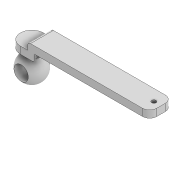
# Autodesk Inventor part: VentilNukleator2
Saved by Autodesk Inventor 2021 (Build 250183000, 183)
## iProperties
Created: 2022-03-14
Part Number: VentilNukleator2
Material: Generisch
Document SubType Name: Modeling
Designer: lukas
Density: 1 g/cm^3
Appearance: Vorgabe
Author: lukas
Autodesk Inventor part; units mm, degrees
ref_plane "YZ Plane" through (0, 0, 0) normal (1, 0, 0) x (0, 1, 0)
ref_plane "XY Plane" through (0, 0, 0) normal (0, 0, 1) x (1, 0, 0)
sketch "Skizze4" plane through (0, 0, 0) normal (0, 0, 1) x (1, 0, 0)
  line L0 (-12.6, 0) -> (12.6, 0) projected
  line L1 (0, -12.6) -> (0, 12.6) projected
  circle A0 centre (0, 0) radius 9
  point P0 (-9, 0)
  point P1 (9, 0)
  dimension "d8" = 18
  constraints: 1 centre point, 1 coincident
  measures "d8" diameter of A0
revolve "Umdrehung1" add sketch "Skizze4" angle 360 about axis through (-10, 0, 0) along (1, 0, 0) picked at (-5.0484, 3.1721) picked at (5.9248, 0.6676) contours A0 L1 L0 | L1 A0 L0
ref_plane "Arbeitsebene1" through (0, 9, 0) normal (0, 1, 0) x (-1, 0, 0)
sketch "Skizze5" plane through (0, 9, 0) normal (0, 1, 0) x (-1, 0, 0)
  circle A0 centre (0, 0) radius 2.5
  dimension "d11" = 5
  constraints: 1 centre point, 1 coincident
  measures "d11" diameter of A0
extrude "Extrusion3" add sketch "Skizze5" along normal mid plane 1
sketch "Skizze6" plane through (0, 9.5, 0) normal (0, 1, 0) x (1, 0, 0)
  circle A0 centre (0, 0) radius 2.5 projected
  circle A1 centre (0, 0) radius 2.5
  dimension "d14" = 5
  constraints: 1 centre point, 1 coincident
  measures "d14" diameter of A1
extrude "Extrusion4" add sketch "Skizze6" along normal blind 2
sketch "Skizze7" plane through (0, 0, 0) normal (0, 0, 1) x (1, 0, 0)
  circle A0 centre (0, 0) radius 5
  dimension "d17" = 10
  constraints: 1 centre point, 1 coincident
  measures "d17" diameter of A0
extrude "Extrusion5" cut sketch "Skizze7" along normal mid plane 20
sketch "Skizze8" plane through (0, 11.5, 0) normal (0, 1, 0) x (1, 0, 0)
  circle A0 centre (0, 0) radius 7.9569
  dimension "d20" = 15.9138
  constraints: 1 centre point, 1 coincident
  measures "d20" diameter of A0
extrude "Extrusion6" add sketch "Skizze8" along normal blind 5
sketch "Skizze9" plane through (0, 0, 0) normal (1, 0, 0) x (0, 1, 0)
  line L0 (16.5, -7.9569) -> (16.5, 7.9569) projected
  line L1 (11.5, -7.9569) -> (11.5, 7.9569) projected
  line L2 (16.5, 7.9569) -> (11.5, 7.9569)
  line L3 (11.5, 7.9569) -> (11.5, -7.9569)
  line L4 (11.5, -7.9569) -> (16.5, -7.9569)
  line L5 (16.5, -7.9569) -> (16.5, 7.9569)
  point P0 (0, 0)
  constraints: 8 end point, 2 parallel, 1 horizontal, 1 perpendicular
extrude "Extrusion7" add sketch "Skizze9" along normal blind 10
sketch "Skizze10" plane through (0, 16.5, 0) normal (0, 1, 0) x (1, 0, 0)
  line L0 (10, 7.9569) -> (10, -7.9569) projected
  line L1 (0, 7.9569) -> (10, 7.9569) projected
  line L2 (10, -7.9569) -> (5, -7.9569)
  line L3 (5, -7.9569) -> (5, 7.9569)
  line L4 (5, 7.9569) -> (10, 7.9569)
  line L5 (10, 7.9569) -> (10, -7.9569)
  point P0 (0, 0)
  dimension "d25" = 5
  constraints: 8 end point, 2 parallel, 1 horizontal, 1 midpoint, 1 perpendicular
  measures "d25" distance between parallel lines of L3 L0
extrude "Extrusion8" add sketch "Skizze10" along normal blind 5
sketch "Skizze11" plane through (10, 0, 0) normal (1, 0, 0) x (0, 0, -1)
  line L0 (7.9569, 11.5) -> (7.9569, 21.5) projected
  line L1 (-7.9569, 11.5) -> (-7.9569, 21.5) projected
  line L2 (7.9569, 21.5) -> (-7.9569, 21.5)
  line L3 (-7.9569, 21.5) -> (-7.9569, 16.5)
  line L4 (-7.9569, 16.5) -> (7.9569, 16.5)
  line L5 (7.9569, 16.5) -> (7.9569, 21.5)
  point P0 (0, 0)
  point P1 (7.9569, 16.5)
  dimension "d28" = 5
  constraints: 8 end point, 2 parallel, 1 horizontal, 1 midpoint, 1 perpendicular
  measures "d28" distance between parallel lines of L4 L2
extrude "Extrusion9" add sketch "Skizze11" along normal blind 80
fillet "Rundung2" radius 2 2 edges at (10, 11.5, 0) (5, 21.5, 0)
fillet "Rundung3" radius 5 2 edges at (90, 19, 7.9569) (90, 19, -7.9569)
sketch "Skizze12" plane through (0, 21.5, 0) normal (0, 1, 0) x (1, 0, 0)
  circle A0 centre (85, 0) radius 1.5
  line L0 (90, 2.9569) -> (90, -2.9569) projected
  point P0 (0, 0)
  dimension "d33" = 3
  dimension "d34" = 5
  constraints: 1 centre point
  measures "d33" diameter of A0
  measures "d34" distance from line of L0 A0.centre
extrude "Extrusion10" cut sketch "Skizze12" against normal blind 5
